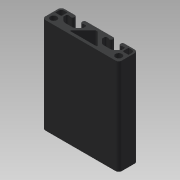
# Autodesk Inventor part: 40-8020.dxf
Saved by Autodesk Inventor 2013 (Build 170138000, 138)
## iProperties
Company: 80/20 Inc.
Created: 2014-04-23
Part Number: 40-8020.dxf
Material: Generic
Document SubType Name: Modeling
Designer: Ross Bowman
Density: 1 g/cm^3
Engineer: Ross Bowman
Catalog Web Link: 8020.net
Vendor: 80/20 Inc.
Material: 6105-T5 Aluminum
Author: Ross Bowman
Keywords: 80/20 , 8020 , T-Slot , Extrusion
Autodesk Inventor part; units mm, degrees
ref_plane "YZ Plane" through (0, 0, 0) normal (1, 0, 0) x (0, 1, 0)
ref_plane "XZ Plane" through (0, 0, 0) normal (0, 1, 0) x (-1, 0, 0)
ref_plane "XY Plane" through (0, 0, 0) normal (0, 0, 1) x (1, 0, 0)
sketch "Sketch1" plane through (0, 0, 0) normal (0, 0, 1) x (1, 0, 0)
  circle A0 centre (34.0048, -4) radius 3.4
  line L0 (31.935, 7.7219) -> (31.935, 3.2459)
  arc A1 (32.564, 8.35) -> (31.935, 7.7219) centre (32.5699, 7.7151) ccw
  line L1 (35.5549, 8.35) -> (32.564, 8.35)
  arc A2 (38.35, 5.4968) -> (35.5549, 8.35) centre (35.557, 5.5563) ccw
  line L2 (38.35, 2.5356) -> (38.35, 5.4968)
  arc A3 (37.6808, 1.976) -> (38.35, 2.5356) centre (37.7194, 2.6098) ccw
  line L3 (33.2048, 1.976) -> (37.6808, 1.976)
  arc A4 (31.935, 3.2459) -> (33.2048, 1.976) centre (33.2048, 3.2459) ccw
  line L4 (-13.4502, -6.9544) -> (13.4502, -6.9544)
  arc A5 (-13.8991, -5.8705) -> (-13.4502, -6.9544) centre (-13.4502, -6.3195) ccw
  line L5 (-1.2578, 6.7693) -> (-13.8991, -5.8705)
  arc A6 (-0.8088, 6.9553) -> (-1.2578, 6.7693) centre (-0.8088, 6.3203) ccw
  line L6 (0.8088, 6.9553) -> (-0.8088, 6.9553)
  arc A7 (1.2578, 6.7693) -> (0.8088, 6.9553) centre (0.8088, 6.3203) ccw
  line L7 (13.8991, -5.8705) -> (1.2578, 6.7693)
  arc A8 (13.4502, -6.9544) -> (13.8991, -5.8705) centre (13.4502, -6.3195) ccw
  line L8 (-37.7151, 1.9604) -> (-33.2048, 1.9604)
  arc A9 (-38.35, 2.5953) -> (-37.7151, 1.9604) centre (-37.7151, 2.5953) ccw
  line L9 (-38.35, 5.5571) -> (-38.35, 2.5953)
  arc A10 (-35.4935, 8.35) -> (-38.35, 5.5571) centre (-35.5563, 5.5571) ccw
  line L10 (-32.5699, 8.35) -> (-35.4935, 8.35)
  arc A11 (-31.935, 7.7151) -> (-32.5699, 8.35) centre (-32.5699, 7.7151) ccw
  line L11 (-31.935, 3.2302) -> (-31.935, 7.7151)
  arc A12 (-33.2048, 1.9604) -> (-31.935, 3.2302) centre (-33.2048, 3.2302) ccw
  circle A13 centre (-34.0048, -4) radius 3.4
  line L12 (13.2285, 5.9365) -> (14.3654, 5.9365)
  arc A14 (14.3654, 5.9365) -> (15.94, 7.5111) centre (14.3654, 7.5111) ccw
  line L13 (15.94, 7.5111) -> (15.94, 8.4254)
  arc A15 (15.94, 8.4254) -> (14.5525, 10) centre (14.3654, 8.4365) ccw
  line L14 (14.5525, 10) -> (-14.3654, 10)
  arc A16 (-14.3654, 10) -> (-15.94, 8.4254) centre (-14.3654, 8.4254) ccw
  line L15 (-15.94, 8.4254) -> (-15.94, 7.5111)
  arc A17 (-15.94, 7.5111) -> (-14.3654, 5.9365) centre (-14.3654, 7.5111) ccw
  line L16 (-14.3654, 5.9365) -> (-13.2285, 5.9365)
  line L17 (-13.2285, 5.9365) -> (-13.2285, 6.4054)
  line L18 (-13.2285, 6.4054) -> (-10.9848, 6.4054)
  arc A18 (-9.715, 5.1355) -> (-10.9848, 6.4054) centre (-10.9848, 5.1355) ccw
  line L19 (-9.715, 5.1355) -> (-9.715, 2.6208)
  arc A19 (-9.9753, 1.9923) -> (-9.715, 2.6208) centre (-10.6039, 2.6208) ccw
  line L20 (-9.9753, 1.9923) -> (-12.8764, -0.9089)
  arc A20 (-16.2347, -2.3) -> (-12.8764, -0.9089) centre (-16.2347, 2.4492) ccw
  line L21 (-16.2347, -2.3) -> (-23.5072, -2.3)
  arc A21 (-26.8655, -0.9089) -> (-23.5072, -2.3) centre (-23.5072, 2.4492) ccw
  line L22 (-26.8655, -0.9089) -> (-30.0247, 2.2504)
  arc A22 (-30.285, 2.879) -> (-30.0247, 2.2504) centre (-29.3961, 2.879) ccw
  line L23 (-30.285, 2.879) -> (-30.285, 5.1355)
  arc A23 (-29.0152, 6.4054) -> (-30.285, 5.1355) centre (-29.0152, 5.1355) ccw
  line L24 (-29.0152, 6.4054) -> (-26.8986, 6.4054)
  line L25 (-26.8986, 6.4054) -> (-26.8986, 5.9365)
  line L26 (-26.8986, 5.9365) -> (-25.7617, 5.9365)
  arc A24 (-25.7617, 5.9365) -> (-24.06, 7.506) centre (-25.6346, 7.506) ccw
  line L27 (-24.06, 7.506) -> (-24.06, 8.4203)
  arc A25 (-24.06, 8.4203) -> (-25.7617, 10) centre (-25.6441, 8.4203) ccw
  line L28 (-25.7617, 10) -> (-36.8282, 10)
  arc A26 (-36.8282, 10) -> (-40, 6.8282) centre (-36.8282, 6.8282) ccw
  line L29 (-40, 6.8282) -> (-40, -6.8282)
  arc A27 (-40, -6.8282) -> (-36.8282, -10) centre (-36.8282, -6.8282) ccw
  line L30 (-36.8282, -10) -> (36.8254, -10)
  arc A28 (36.8254, -10) -> (40, -6.8282) centre (36.8254, -6.8254) ccw
  line L31 (40, -6.8282) -> (40, 6.8282)
  arc A29 (40, 6.8282) -> (36.8854, 10) centre (36.8254, 6.826) ccw
  line L32 (36.8854, 10) -> (25.4475, 10)
  arc A30 (25.4475, 10) -> (24.06, 8.4254) centre (25.6346, 8.4365) ccw
  line L33 (24.06, 8.4254) -> (24.06, 7.5111)
  arc A31 (24.06, 7.5111) -> (25.6346, 5.9365) centre (25.6346, 7.5111) ccw
  line L34 (25.6346, 5.9365) -> (26.7715, 5.9365)
  line L35 (26.7715, 5.9365) -> (26.7715, 6.6606)
  line L36 (26.7715, 6.6606) -> (29.0152, 6.6606)
  arc A32 (30.285, 5.3908) -> (29.0152, 6.6606) centre (29.0152, 5.3908) ccw
  line L37 (30.285, 5.3908) -> (30.285, 3.1342)
  arc A33 (30.0247, 2.2504) -> (30.285, 3.1342) centre (29.4256, 2.9071) ccw
  line L38 (30.0247, 2.2504) -> (26.8655, -0.9089)
  arc A34 (23.5072, -2.3) -> (26.8655, -0.9089) centre (23.5072, 2.4492) ccw
  line L39 (23.5072, -2.3) -> (16.4928, -2.3)
  arc A35 (13.1345, -0.6536) -> (16.4928, -2.3) centre (16.7353, 2.443) ccw
  line L40 (13.1345, -0.6536) -> (9.9753, 2.5057)
  arc A36 (9.715, 3.1342) -> (9.9753, 2.5057) centre (10.6039, 3.1342) ccw
  line L41 (9.715, 3.1342) -> (9.715, 5.3908)
  arc A37 (10.9848, 6.6606) -> (9.715, 5.3908) centre (10.9848, 5.3908) ccw
  line L42 (10.9848, 6.6606) -> (13.2285, 6.6606)
  line L43 (13.2285, 6.6606) -> (13.2285, 5.9365)
  point P0 (0, 0)
  constraints: 88 end point, 72 point on circle, 38 centre point
extrude "Extrusion1" add sketch "Sketch1" against normal blind 100
body "Solid1"
